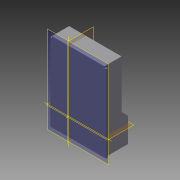
# Autodesk Inventor part: batteri
Saved by Autodesk Inventor 2015 (Build 190159000, 159)
## iProperties
Created: 2015-12-13
Part Number: batteri
Material: Generic
Document SubType Name: Modeling
Designer: abberik
Density: 1 g/cm^3
Appearance: Default
Author: abberik
Autodesk Inventor part; units mm, degrees
sketch "Sketch1" plane through (0, 0, 0) normal (0, 1, 0) x (-1, 0, 0)
  line L0 (22.3723, -21.9307) -> (-45.6277, -21.9307)
  line L1 (-45.6277, -21.9307) -> (-45.6277, 74.5693)
  line L2 (-45.6277, 74.5693) -> (22.3723, 74.5693)
  line L3 (22.3723, 74.5693) -> (22.3723, -21.9307)
  point P0 (0, 0)
  dimension "d0" = 68
  dimension "d1" = 96.5
  constraints: 8 end point, 2 parallel, 1 horizontal, 1 perpendicular
  measures "d0" distance between parallel lines of L1 L3
  measures "d1" distance between parallel lines of L0 L2
extrude "Extrusion1" add sketch "Sketch1" along normal blind 2
sketch "Sketch3" plane through (0, 2, 0) normal (0, 1, 0) x (1, 0, 0)
  line L0 (-20.3723, 21.9307) -> (43.6277, 21.9307)
  line L1 (43.6277, 21.9307) -> (43.6277, -72.5693)
  line L2 (-20.3723, -72.5693) -> (-20.3723, 21.9307)
  line L3 (45.6277, 21.9307) -> (-22.3723, 21.9307) projected
  line L4 (-22.3723, 21.9307) -> (-22.3723, -74.5693) projected
  line L5 (-22.3723, -74.5693) -> (45.6277, -74.5693) projected
  line L6 (45.6277, -74.5693) -> (45.6277, 21.9307) projected
  line L7 (-20.3723, -72.5693) -> (-20.3723, -74.5693)
  line L8 (-22.3723, -74.5693) -> (45.6277, -74.5693) projected
  line L9 (43.6277, -74.5693) -> (43.6277, -72.5693)
  line L10 (-18.3723, -72.5693) -> (41.6277, -72.5693)
  line L11 (41.6277, -72.5693) -> (41.6277, 21.9307)
  line L12 (41.6277, 21.9307) -> (-18.3723, 21.9307)
  line L13 (-18.3723, 21.9307) -> (-18.3723, -72.5693)
  point P0 (0, 0)
  dimension "d4" = 0
  dimension "d5" = 2
  dimension "d7" = 2
  dimension "d8" = 0
  dimension "d9" = 2
  dimension "d10" = 2
  dimension "d11" = 2
  constraints: 18 end point, 4 perpendicular, 3 parallel, 2 horizontal, 2 point on line
  measures "d4" distance between parallel lines of L3 L0
  measures "d5" distance between parallel lines of L6 L1
  measures "d7" distance between parallel lines of L4 L2
  measures "d8" distance between parallel lines of L0 L12
  measures "d9" distance between parallel lines of L2 L13
  measures "d10" distance between parallel lines of L1 L11
  measures "d11" distance between parallel lines of L5 L10
extrude "Extrusion2" add sketch "Sketch3" along normal blind 25 contours L0 L13 L10 L11 L1 L9 L5 L7 L2
sketch "Sketch4" plane through (0, 27, 0) normal (0, 1, 0) x (1, 0, 0)
  line L0 (41.6277, 21.9307) -> (41.6277, -72.5693) projected
  line L1 (41.6277, -72.5693) -> (-18.3723, -72.5693) projected
  line L2 (-18.3723, -72.5693) -> (-18.3723, 21.9307) projected
  line L3 (-18.3723, 21.9307) -> (-20.3723, 21.9307) projected
  line L4 (-20.3723, 21.9307) -> (-20.3723, -74.5693) projected
  line L5 (-20.3723, -74.5693) -> (43.6277, -74.5693) projected
  line L6 (43.6277, -74.5693) -> (43.6277, 21.9307) projected
  line L7 (43.6277, 21.9307) -> (41.6277, 21.9307) projected
  line L8 (-20.3723, 21.9307) -> (43.6277, 21.9307)
  line L9 (43.6277, 21.9307) -> (43.6277, -74.5693)
  line L10 (43.6277, -74.5693) -> (-20.3723, -74.5693)
  line L11 (-20.3723, -74.5693) -> (-20.3723, 21.9307)
  point P0 (0, 0)
  constraints: 8 end point, 2 parallel, 1 horizontal, 1 perpendicular
extrude "Extrusion3" add sketch "Sketch4" along normal blind 2
sketch "Sketch5" plane through (0, 2, 0) normal (0, 1, 0) x (1, 0, 0)
  line L0 (43.6277, 21.9307) -> (43.6277, -74.5693) projected
  line L1 (43.6277, -74.5693) -> (45.6277, -74.5693) projected
  line L2 (45.6277, -74.5693) -> (45.6277, 21.9307) projected
  line L3 (45.6277, 21.9307) -> (43.6277, 21.9307) projected
  line L4 (-20.3723, -74.5693) -> (-20.3723, 21.9307) projected
  line L5 (-20.3723, 21.9307) -> (-22.3723, 21.9307) projected
  line L6 (-22.3723, 21.9307) -> (-22.3723, -74.5693) projected
  line L7 (-22.3723, -74.5693) -> (-20.3723, -74.5693) projected
  line L8 (-22.3723, -74.5693) -> (-20.3723, -74.5693)
  line L9 (-20.3723, -74.5693) -> (-20.3723, -72.5693)
  line L10 (-20.3723, -72.5693) -> (-22.3723, -72.5693)
  line L11 (-22.3723, -72.5693) -> (-22.3723, -74.5693)
  line L12 (43.6277, -74.5693) -> (43.6277, 21.9307) projected
  line L13 (45.6277, -74.5693) -> (43.6277, -74.5693)
  line L14 (43.6277, -74.5693) -> (43.6277, -72.5693)
  line L15 (43.6277, -72.5693) -> (45.6277, -72.5693)
  line L16 (45.6277, -72.5693) -> (45.6277, -74.5693)
  point P0 (0, 0)
  dimension "d16" = 2
  dimension "d17" = 2
  constraints: 16 end point, 4 parallel, 2 horizontal, 2 perpendicular, 1 point on line
  measures "d16" distance of L10.end L9.end
  measures "d17" distance of L9.end L8.end
extrude "Extrusion4" cut sketch "Sketch5" against normal blind 2 contours L15 L2 L1 L0 | L7 L6 L10 L4
sketch "Sketch6" plane through (-20.3723, 0, 74.5693) normal (-1, 0, 0) x (0, 0, 1)
  line L0 (-96.5, 29) -> (-69.5, 29)
  line L1 (-96.5, 29) -> (0, 29) projected
  line L2 (0, 0) -> (0, 29) projected
  line L3 (0, 19) -> (-59.5, 19)
  line L4 (-69.5, 29) -> (-59.5, 19)
  line L5 (-69.5, 29) -> (-55.3579, 29) construction
  line L6 (-69.5, 29) -> (0, 29)
  line L7 (0, 29) -> (0, 19)
  point P0 (-74.5693, 0)
  dimension "d20" = 27
  dimension "d21" = 10
  dimension "d22" = 45
  constraints: 12 end point, 3 horizontal, 2 point on line, 1 collinear, 1 equal length
  measures "d20" distance of L0.start L0.end
  measures "d21" distance between parallel lines of L1 L3
  measures "d22" angle of L4 L5
extrude "Extrusion5" cut sketch "Sketch6" against normal up to next
sketch "Sketch7" plane through (-20.3723, 2, -21.9307) normal (-1, 0, 0) x (0, 0, 1)
  line L0 (37, 17) -> (27, 27) projected
  line L1 (96.5, 17) -> (37, 17) projected
  line L2 (29.8284, 27) -> (37.8284, 19)
  line L3 (37.8284, 19) -> (96.5, 19)
  line L4 (27, 27) -> (29.8284, 27)
  line L5 (96.5, 17) -> (96.5, 19)
  point P0 (21.9307, -2)
  dimension "d25" = 2
  constraints: 8 end point, 1 horizontal, 1 vertical
  measures "d25" distance between parallel lines of L0 L2
extrude "Extrusion6" add sketch "Sketch7" against normal up to surface (64 mm away)
sketch "Sketch13" plane through (-20.3723, 2, -21.9307) normal (-1, 0, 0) x (0, 0, 1)
  line L0 (2.109, 2.4048) -> (12.109, 2.4048)
  line L1 (12.109, 2.4048) -> (12.109, 17.4048)
  line L2 (12.109, 17.4048) -> (2.109, 17.4048)
  line L3 (2.109, 17.4048) -> (2.109, 2.4048)
  point P0 (21.9307, -2)
  dimension "d46" = 10
  dimension "d47" = 15
  constraints: 8 end point, 2 parallel, 1 horizontal, 1 perpendicular
  measures "d46" distance of L2.end L1.end
  measures "d47" distance of L1.end L0.end
extrude "Extrusion7" cut sketch "Sketch13" against normal blind 2
body "Solid1"
